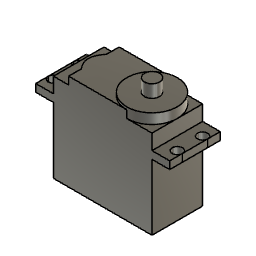
actual acutator v0 v1 (Autodesk Fusion 360 design; units mm, degrees)
Autodesk Fusion 360 part; units mm, degrees
note: some values were not read from the file. Set by a fixed rule: which sketch regions a step uses.
sketch "Sketch1" plane through (0, 0, 0) normal (0, 1, 0) x (1, 0, 0)
  line L0 (0, 0) -> (53, 0)
  line L1 (53, 0) -> (53, -39)
  line L2 (53, -39) -> (0, -39)
  line L3 (0, -39) -> (0, 0)
  dimension "d1" = 53
  dimension "d2" = 39
  constraint horizontal L0
  constraint vertical L1
  constraint horizontal L2
  constraint vertical L3
  constraint coincident L0.start L3.end
  measures "d1" distance of L0.start L0.end
  measures "d2" distance of L0.start L2.end
extrude "Extrude1" add sketch "Sketch1" along normal blind 20
sketch "Sketch2" plane through (0, 0, 39) normal (0, 0, 1) x (-1, 0, 0)
  line L0 (0, 0) -> (-53, 0)
  line L1 (-53, 0) -> (-53, -20)
  line L2 (-53, -20) -> (0, -20)
  line L3 (0, -20) -> (0, 0)
  line L4 (0, -20) -> (-7, -20)
  line L5 (-7, -20) -> (-7, 0)
  line L6 (-7, 0) -> (0, 0)
  line L7 (0, 0) -> (0, -20)
  line L8 (-53, -20) -> (-46, -20)
  line L9 (-46, -20) -> (-46, 0)
  line L10 (-46, 0) -> (-53, 0)
  line L11 (-53, 0) -> (-53, -20)
  dimension "d5" = 7
  dimension "d6" = 7
  constraint horizontal L4
  constraint vertical L5
  constraint horizontal L6
  constraint vertical L7
  constraint coincident L2.end L3.start
  constraint horizontal L8
  constraint vertical L9
  constraint horizontal L10
  constraint vertical L11
  constraint coincident L0 L9.end
  constraint coincident L1.end L2.start
  measures "d5" distance of L2.end L4.end
  measures "d6" distance of L1.end L8.end
extrude "Extrude2" cut sketch "Sketch2" against normal blind 10 contours L0 L2 L3 L4 L5 L6 L7 | L0 L1 L2 L8 L9 L10 L11
sketch "Sketch3" plane through (0, 0, 0) normal (0, 0, -1) x (1, 0, 0)
  line L0 (53, 0) -> (0, 0)
  line L1 (0, 0) -> (0, -20)
  line L2 (0, -20) -> (53, -20)
  line L3 (53, -20) -> (53, 0)
  line L4 (0, 0) -> (7, 0)
  line L5 (7, 0) -> (7, -20)
  line L6 (7, -20) -> (0, -20)
  line L7 (0, -20) -> (0, 0)
  line L8 (53, 0) -> (46, 0)
  line L9 (46, 0) -> (46, -20)
  line L10 (46, -20) -> (53, -20)
  line L11 (53, -20) -> (53, 0)
  dimension "d9" = 7
  dimension "d10" = 7
  constraint horizontal L4
  constraint vertical L5
  constraint horizontal L6
  constraint vertical L7
  constraint coincident L0.end L1.start
  constraint horizontal L8
  constraint vertical L9
  constraint horizontal L10
  constraint vertical L11
  constraint coincident L0.start L3.end
  measures "d9" distance of L0.end L4.end
  measures "d10" distance of L0.start L8.end
extrude "Extrude3" cut sketch "Sketch3" against normal blind 26 contours L0 L2 L3 L8 L9 L10 L11 | L0 L1 L2 L4 L5 L6 L7
sketch "Sketch4" plane through (0, 0, 39) normal (0, 0, 1) x (-1, 0, 0)
  line L0 (-7, -20) -> (-7, 0)
  line L1 (-7, 0) -> (-46, 0)
  line L2 (-46, 0) -> (-46, -20)
  line L3 (-46, -20) -> (-7, -20)
  line L4 (-7, -20) -> (-13, -20)
  line L5 (-13, -20) -> (-13, 0)
  line L6 (-13, 0) -> (-7, 0)
  line L7 (-7, 0) -> (-7, -20)
  circle A0 centre (-36, -10) radius 10
  circle A1 centre (-36, -10) radius 6.5
  circle A2 centre (-36, -10) radius 3
  spline S0 degree 5 poles (-13, -15.0203) (-12.838, -14.8194) (-12.5281, -14.4176) (-12.1057, -13.8151) (-11.6287, -13.012) (-11.1861, -12.0086) (-10.9107, -11.0057) (-10.8163, -10.0034) (-10.9104, -9.0017) (-11.1856, -8.0005) (-11.6282, -6.9998) (-12.1053, -6.1997) (-12.5279, -5.5998) (-12.8379, -5.1999) (-13, -5) knots 0 0 0 0 0 0 0.1 0.2 0.3 0.4 0.5 0.6 0.7 0.8 0.9 1 1 1 1 1 1
  point P0 (-13, -10)
  point P1 (-13, -15.0203)
  point P2 (-13, -5)
  point P3 (-10.8633, -10)
  dimension "d13" = 6
  dimension "d14" = 20
  dimension "d15" = 13
  dimension "d16" = 6
  constraint horizontal L4
  constraint vertical L5
  constraint horizontal L6
  constraint vertical L7
  constraint coincident L0.start L3.end
  constraint tangent L3 A0
  constraint tangent L2 A0
  constraint tangent L1 A0
  constraint concentric A0 A1
  constraint concentric A1 A2
  constraint midpoint L5 P0
  constraint coincident L5 P1
  constraint coincident L5 P2
  constraint coincident P2 S0.end
  measures "d13" distance of L0.start L4.end
  measures "d14" distance of L0.start L0.end
  measures "d15" diameter of A1
  measures "d16" diameter of A2
extrude "Extrude4" cut sketch "Sketch4" against normal blind 4 contours L0 L1 L3 L4 L5 L6 L7 S0 | L2 L3 A0 | L1 L2 A0
extrude "Extrude5" cut sketch "Sketch4" against normal blind 1 contours L1 L3 L5 A0 | L2 L3 A0 | L5 S0 | L1 L2 A0
extrude "Extrude6" add sketch "Sketch4" along normal blind 5 contours A2
sketch "Sketch5" plane through (0, 0, 29) normal (0, 0, 1) x (-1, 0, 0)
  line L0 (-53, 0) -> (-53, -20)
  line L1 (-53, -20) -> (-46, -20)
  line L2 (-46, -20) -> (-46, 0)
  line L3 (-46, 0) -> (-53, 0)
  line L4 (-53, 0) -> (-51, 0)
  line L5 (-51, 0) -> (-51, -5)
  line L6 (-51, -5) -> (-53, -5)
  line L7 (-53, -5) -> (-53, 0)
  circle A0 centre (-51, -5) radius 2
  line L8 (-53, -20) -> (-51, -20)
  line L9 (-51, -20) -> (-51, -15)
  line L10 (-51, -15) -> (-53, -15)
  line L11 (-53, -15) -> (-53, -20)
  circle A1 centre (-51, -15) radius 2
  dimension "d23" = 2
  dimension "d24" = 5
  dimension "d25" = 4
  dimension "d26" = 2
  dimension "d27" = 5
  dimension "d28" = 4
  constraint horizontal L4
  constraint vertical L5
  constraint horizontal L6
  constraint vertical L7
  constraint coincident L0.start L3.end
  constraint coincident L5.end L6.start
  constraint horizontal L8
  constraint vertical L9
  constraint horizontal L10
  constraint vertical L11
  constraint coincident L0.end L1.start
  constraint coincident L9.end L10.start
  measures "d23" distance of L0.start L4.end
  measures "d24" distance of L0.start L6.end
  measures "d25" diameter of A0
  measures "d26" distance of L0.end L8.end
  measures "d27" distance of L0.end L10.end
  measures "d28" diameter of A1
extrude "Extrude7" cut sketch "Sketch5" against normal blind 3 contours L5 L6 A0 | L5 L6 A0 | L9 L10 A1 | L9 L10 A1
ref_plane "WorkPlane1" through (26.5, 0, 0) normal (1, 0, 0) x (0, 1, 0)
mirror "Mirror1" about plane through (26.5, 0, 0) normal (1, 0, 0) of "Extrude7"
